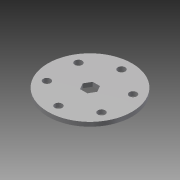
# Autodesk Inventor part: Hub v1
Saved by Autodesk Inventor 2013 (Build 170138000, 138)
## iProperties
Created: 2013-01-16
Part Number: Hub v1
Material: Steel
Document SubType Name: Modeling
Designer: actoennies
Mass: 71.7827 g
Surface Area: 68.6768 cm^2
Volume: 9.14429 cm^3
Density: 7.85 g/cm^3
Author: actoennies
Autodesk Inventor part; units mm, degrees
ref_plane "YZ Plane" through (0, 0, 0) normal (1, 0, 0) x (0, 1, 0)
ref_plane "XZ Plane" through (0, 0, 0) normal (0, 1, 0) x (-1, 0, 0)
ref_plane "XY Plane" through (0, 0, 0) normal (0, 0, 1) x (1, 0, 0)
sketch "Sketch1" plane through (0, 0, 0) normal (0, 1, 0) x (-1, 0, 0)
  circle A0 centre (0, 0) radius 31.75
  circle A1 centre (0, -23.8125) radius 2.794
  circle A2 centre (20.6222, -11.9063) radius 2.794
  circle A3 centre (20.6222, 11.9062) radius 2.794
  circle A4 centre (0, 23.8125) radius 2.794
  circle A5 centre (-20.6222, 11.9062) radius 2.794
  circle A6 centre (-20.6222, -11.9063) radius 2.794
  line L0 (2.7496, 4.7625) -> (5.4993, 0)
  line L1 (5.4993, 0) -> (2.7496, -4.7625)
  line L2 (2.7496, -4.7625) -> (-2.7496, -4.7625)
  line L3 (-2.7496, -4.7625) -> (-5.4993, 0)
  line L4 (-5.4993, 0) -> (-2.7496, 4.7625)
  line L5 (-2.7496, 4.7625) -> (2.7496, 4.7625)
  line L6 (0, 0) -> (0, -23.8125) construction
  dimension "d5" = 5.588
  dimension "d9" = 360
  dimension "d22" = 9.525
  dimension "d25" = 23.8125
  constraints: 14 end point, 7 centre point, 1 coincident, 1 perpendicular, 1 vertical, 27 other
  measures "d5" diameter of A1
  measures "d22" distance between parallel lines of L2 L5
  measures "d25" distance of A0.centre L6.end
extrude "Extrusion3" add sketch "Sketch1" along normal blind 3.175
body "Solid3"
